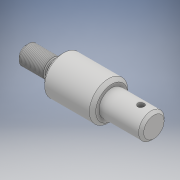
# Autodesk Inventor part: Вал
Saved by Autodesk Inventor 2018 (Build 220112000, 112)
## iProperties
Part Number: Вал
Material: Типовые
Document SubType Name: Modeling
Designer: 2000
Density: 1 g/cm^3
Appearance: По умолчанию
Mass: 41.4825 g
Surface Area: 85.4136 cm^2
Volume: 41.4825 cm^3
Author: 2000
Autodesk Inventor part; units mm, degrees
ref_plane "YZ Plane" through (0, 0, 0) normal (1, 0, 0) x (0, 1, 0)
ref_plane "XY Plane" through (0, 0, 0) normal (0, 0, 1) x (1, 0, 0)
sketch "Эскиз1" plane through (0, 0, 0) normal (0, 0, 1) x (1, 0, 0)
  line L0 (0, 0) -> (0, 7.5)
  line L1 (22.4142, 6.5) -> (25.4, 6.5)
  line L2 (27, 8.1) -> (27, 15)
  line L3 (27, 15) -> (67, 15)
  line L4 (100, 10) -> (100, 0)
  line L5 (100, 0) -> (0, 0)
  line L6 (0, 7.5) -> (21, 7.5)
  line L7 (21, 7.5) -> (21.7071, 6.7929)
  line L8 (100, 10) -> (67, 10)
  line L9 (67, 15) -> (67, 10)
  arc A0 (21.7071, 6.7929) -> (22.4142, 6.5) centre (22.4142, 7.5) ccw
  arc A1 (25.4, 6.5) -> (27, 8.1) centre (25.4, 8.1) ccw
  point P0 (22, 6.5)
  point P1 (27, 6.5)
  point P2 (67, 12.5)
  dimension "d0" = 27
  dimension "d4" = 100
  dimension "d14" = 6.5
  dimension "d21" = 135
  dimension "d22" = 1
  dimension "d23" = 5
  dimension "d26" = 10
  dimension "d27" = 40
  dimension "d28" = 15
  dimension "d70" = 1
  dimension "d71" = 1.6
  constraints: 20 end point, 4 point on circle, 4 point on line, 4 tangent, 2 centre point, 2 horizontal, 2 vertical alignment, 1 horizontal alignment, 1 midpoint, 1 perpendicular, 1 vertical
  measures "d0" horizontal distance of L0.end point (27, 6.5)
  measures "d4" distance of L4.end L0.start
  measures "d14" distance between parallel lines of L5 L1
  measures "d21" angle of L1 L7
  measures "d22" distance between parallel lines of L1 L6
  measures "d23" distance of point (22, 6.5) point (27, 6.5)
  measures "d26" distance between parallel lines of L8 L5
  measures "d27" distance of L2.end L3.end
  measures "d28" distance between parallel lines of L5 L3
  measures "d70" radius of A0
  measures "d71" radius of A1
revolve "Вращение1" add sketch "Эскиз1" angle 360 about axis through (100, 0, 0) along (-1, 0, 0)
sketch "Эскиз2" plane through (0, 0, 0) normal (0, 0, 1) x (1, 0, 0)
  point P0 (0, 0)
sketch "Эскиз4" plane through (0, 0, 0) normal (0, 0, 1) x (1, 0, 0)
  circle A0 centre (90, 0) radius 2.5
  line L0 (100, -10) -> (100, 10) projected
  point P0 (0, 0)
  dimension "d38" = 10
  dimension "d39" = 5
  dimension "d40" = 90
  constraints: 1 centre point
  measures "d38" distance from line of L0 A0.centre
  measures "d39" diameter of A0
  measures "d40" distance of A0.centre point (0, 0)
extrude "Выдавливание2" cut sketch "Эскиз4" along normal through all both and the other way through all
thread "Резьба1" size "M16x1" class "6g" standard "ISO Metric profile" full length
chamfer "Фаска1" distance 2 angle 45 1 edges at (0, -7.5, 0)
chamfer "Фаска2" distance 2.5 angle 45 1 edges at (67, -15, 0) measured on face at (67, 13.0912, 1.9943)
chamfer "Фаска3" distance 2 angle 45 1 edges at (100, -10, 0) measured on face at (100, -0.4018, -2.9244)
chamfer "Фаска4" distance 2.5 angle 45 1 edges at (27, -15, 0) measured on face at (27, 12.5547, 1.1966)
ref_plane "РабПлоскость1" through (0, 11, 0) normal (0, 1, 0) x (-1, 0, 0)
sketch "Эскиз5" plane through (0, 11, 0) normal (0, 1, 0) x (-1, 0, 0)
  line L0 (-29.5, -15) -> (-29.5, 15) projected
  line L1 (11.4, 0) -> (-68.4, 0) projected
  line L2 (-27, -8.5) -> (-27, 8.5) projected
  arc A0 (-41, -4) -> (-41, 4) centre (-41, 0) ccw
  line L3 (-41, -4) -> (-53, -4)
  arc A1 (-53, 4) -> (-53, -4) centre (-53, 0) ccw
  line L4 (-41, 4) -> (-53, 4)
  point P0 (0, 0)
  dimension "d66" = 10
  dimension "d67" = 20
  dimension "d68" = 8
  dimension "d69" = 4
  constraints: 4 end point, 4 point on circle, 2 centre point, 2 horizontal, 2 point on line, 2 tangent
  measures "d66" distance edge to line of A0 L2
  measures "d68" distance between parallel lines of L4 L3
  measures "d69" radius of A1
extrude "Выдавливание3" cut sketch "Эскиз5" along normal blind 4
